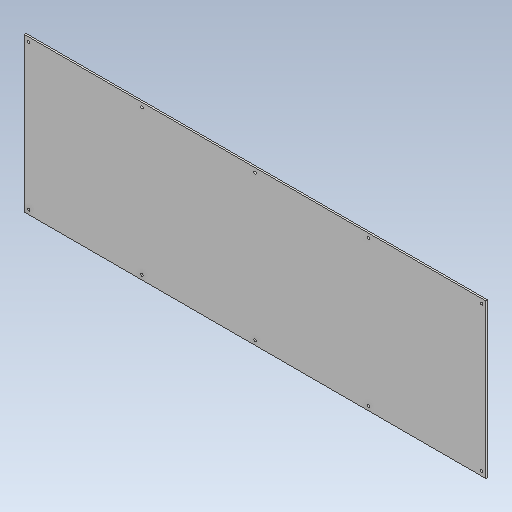
# Autodesk Inventor part: between aluminium and ferrite
Saved by Autodesk Inventor 2021 (Build 250183000, 183)
## iProperties
Created: 2022-01-22
Part Number: between aluminium and ferrite
Material: Generic
Document SubType Name: Modeling
Designer: avan411
Density: 1 g/cm^3
Appearance: Default
Author: avan411
Autodesk Inventor part; units mm, degrees
ref_plane "YZ Plane" through (0, 0, 0) normal (1, 0, 0) x (0, 1, 0)
ref_plane "XZ Plane" through (0, 0, 0) normal (0, 1, 0) x (-1, 0, 0)
ref_plane "XY Plane" through (0, 0, 0) normal (0, 0, 1) x (1, 0, 0)
sketch "Sketch1" plane through (0, 0, 0) normal (0, 0, 1) x (1, 0, 0)
  line L0 (525, 175) -> (-525, 175) projected
  line L1 (525, -175) -> (-525, -175) projected
  line L2 (-525, 175) -> (-525, -175) projected
  line L3 (525, -175) -> (525, 175) projected
  circle A0 centre (515, 165) radius 3 projected
  line L4 (525, -175) -> (-525, -175) projected
  line L5 (-525, -175) -> (-525, 175) projected
  line L6 (-525, 175) -> (525, 175) projected
  line L7 (525, 175) -> (525, -175) projected
  circle A1 centre (-515, 165) radius 3 projected
  circle A2 centre (257.5, 165) radius 3 projected
  circle A3 centre (-515, -165) radius 3 projected
  circle A4 centre (-257.5, -165) radius 3 projected
  circle A5 centre (0, -165) radius 3 projected
  circle A6 centre (257.5, -165) radius 3 projected
  circle A7 centre (515, -165) radius 3 projected
  circle A8 centre (-257.5, 165) radius 3 projected
  circle A9 centre (0, 165) radius 3 projected
  circle A10 centre (515, 165) radius 3 projected
  arc A11 (434.5, 36.45) -> (475.35, 77.3) centre (434.5, 77.3) ccw projected
  line L8 (434.5, 36.45) -> (0, 36.45) projected
  line L9 (0, 36.45) -> (0, 32.15) projected
  line L10 (0, 32.15) -> (434.5, 32.15) projected
  arc A12 (434.5, 32.15) -> (479.65, 77.3) centre (434.5, 77.3) ccw projected
  line L11 (479.65, 77.3) -> (479.65, 85.5) projected
  arc A13 (479.65, 85.5) -> (434.5, 130.65) centre (434.5, 85.5) ccw projected
  line L12 (434.5, 130.65) -> (-434.5, 130.65) projected
  arc A14 (-434.5, 130.65) -> (-479.65, 85.5) centre (-434.5, 85.5) ccw projected
  line L13 (-479.65, 85.5) -> (-479.65, 65.8667) projected
  arc A15 (-479.65, 65.8667) -> (-434.5, 20.7167) centre (-434.5, 65.8667) ccw projected
  line L14 (-434.5, 20.7167) -> (445.75, 20.7167) projected
  arc A16 (445.75, 20.7167) -> (490.9, 65.8667) centre (445.75, 65.8667) ccw projected
  line L15 (490.9, 65.8667) -> (490.9, 96.25) projected
  arc A17 (490.9, 96.25) -> (445.75, 141.4) centre (445.75, 96.25) ccw projected
  line L16 (445.75, 141.4) -> (-445.75, 141.4) projected
  arc A18 (-445.75, 141.4) -> (-490.9, 96.25) centre (-445.75, 96.25) ccw projected
  line L17 (-490.9, 96.25) -> (-490.9, 54.4333) projected
  arc A19 (-490.9, 54.4333) -> (-445.75, 9.2833) centre (-445.75, 54.4333) ccw projected
  line L18 (-445.75, 9.2833) -> (457, 9.2833) projected
  arc A20 (457, 9.2833) -> (502.15, 54.4333) centre (457, 54.4333) ccw projected
  line L19 (502.15, 54.4333) -> (502.15, 107) projected
  arc A21 (502.15, 107) -> (457, 152.15) centre (457, 107) ccw projected
  line L20 (457, 152.15) -> (-457, 152.15) projected
  arc A22 (-457, 152.15) -> (-502.15, 107) centre (-457, 107) ccw projected
  line L21 (-502.15, 107) -> (-502.15, 43) projected
  arc A23 (-502.15, 43) -> (-457, -2.15) centre (-457, 43) ccw projected
  line L22 (-457, -2.15) -> (457, -2.15) projected
  arc A24 (497.85, -43) -> (457, -2.15) centre (457, -43) ccw projected
  line L23 (497.85, -43) -> (497.85, -107) projected
  arc A25 (457, -147.85) -> (497.85, -107) centre (457, -107) ccw projected
  line L24 (457, -147.85) -> (-457, -147.85) projected
  arc A26 (-497.85, -107) -> (-457, -147.85) centre (-457, -107) ccw projected
  line L25 (-497.85, -107) -> (-497.85, -54.4333) projected
  arc A27 (-457, -13.5833) -> (-497.85, -54.4333) centre (-457, -54.4333) ccw projected
  line L26 (-457, -13.5833) -> (445.75, -13.5833) projected
  arc A28 (486.6, -54.4333) -> (445.75, -13.5833) centre (445.75, -54.4333) ccw projected
  line L27 (486.6, -54.4333) -> (486.6, -96.25) projected
  arc A29 (445.75, -137.1) -> (486.6, -96.25) centre (445.75, -96.25) ccw projected
  line L28 (445.75, -137.1) -> (-445.75, -137.1) projected
  arc A30 (-486.6, -96.25) -> (-445.75, -137.1) centre (-445.75, -96.25) ccw projected
  line L29 (-486.6, -96.25) -> (-486.6, -65.8667) projected
  arc A31 (-445.75, -25.0167) -> (-486.6, -65.8667) centre (-445.75, -65.8667) ccw projected
  line L30 (-445.75, -25.0167) -> (434.5, -25.0167) projected
  arc A32 (475.35, -65.8667) -> (434.5, -25.0167) centre (434.5, -65.8667) ccw projected
  line L31 (475.35, -65.8667) -> (475.35, -85.5) projected
  arc A33 (434.5, -126.35) -> (475.35, -85.5) centre (434.5, -85.5) ccw projected
  line L32 (434.5, -126.35) -> (-434.5, -126.35) projected
  arc A34 (-475.35, -85.5) -> (-434.5, -126.35) centre (-434.5, -85.5) ccw projected
  line L33 (-475.35, -85.5) -> (-475.35, -77.3) projected
  arc A35 (-434.5, -36.45) -> (-475.35, -77.3) centre (-434.5, -77.3) ccw projected
  line L34 (-434.5, -36.45) -> (0, -36.45) projected
  line L35 (0, -36.45) -> (0, -32.15) projected
  line L36 (0, -32.15) -> (-434.5, -32.15) projected
  arc A36 (-434.5, -32.15) -> (-479.65, -77.3) centre (-434.5, -77.3) ccw projected
  line L37 (-479.65, -77.3) -> (-479.65, -85.5) projected
  arc A37 (-479.65, -85.5) -> (-434.5, -130.65) centre (-434.5, -85.5) ccw projected
  line L38 (-434.5, -130.65) -> (434.5, -130.65) projected
  arc A38 (434.5, -130.65) -> (479.65, -85.5) centre (434.5, -85.5) ccw projected
  line L39 (479.65, -85.5) -> (479.65, -65.8667) projected
  arc A39 (479.65, -65.8667) -> (434.5, -20.7167) centre (434.5, -65.8667) ccw projected
  line L40 (434.5, -20.7167) -> (-445.75, -20.7167) projected
  arc A40 (-445.75, -20.7167) -> (-490.9, -65.8667) centre (-445.75, -65.8667) ccw projected
  line L41 (-490.9, -65.8667) -> (-490.9, -96.25) projected
  arc A41 (-490.9, -96.25) -> (-445.75, -141.4) centre (-445.75, -96.25) ccw projected
  line L42 (-445.75, -141.4) -> (445.75, -141.4) projected
  arc A42 (445.75, -141.4) -> (490.9, -96.25) centre (445.75, -96.25) ccw projected
  line L43 (490.9, -96.25) -> (490.9, -54.4333) projected
  arc A43 (490.9, -54.4333) -> (445.75, -9.2833) centre (445.75, -54.4333) ccw projected
  line L44 (445.75, -9.2833) -> (-457, -9.2833) projected
  arc A44 (-457, -9.2833) -> (-502.15, -54.4333) centre (-457, -54.4333) ccw projected
  line L45 (-502.15, -54.4333) -> (-502.15, -107) projected
  arc A45 (-502.15, -107) -> (-457, -152.15) centre (-457, -107) ccw projected
  line L46 (-457, -152.15) -> (457, -152.15) projected
  arc A46 (457, -152.15) -> (502.15, -107) centre (457, -107) ccw projected
  line L47 (502.15, -107) -> (502.15, -43) projected
  arc A47 (502.15, -43) -> (457, 2.15) centre (457, -43) ccw projected
  line L48 (457, 2.15) -> (-457, 2.15) projected
  arc A48 (-497.85, 43) -> (-457, 2.15) centre (-457, 43) ccw projected
  line L49 (-497.85, 43) -> (-497.85, 107) projected
  arc A49 (-457, 147.85) -> (-497.85, 107) centre (-457, 107) ccw projected
  line L50 (-457, 147.85) -> (457, 147.85) projected
  arc A50 (497.85, 107) -> (457, 147.85) centre (457, 107) ccw projected
  line L51 (497.85, 107) -> (497.85, 54.4333) projected
  arc A51 (457, 13.5833) -> (497.85, 54.4333) centre (457, 54.4333) ccw projected
  line L52 (457, 13.5833) -> (-445.75, 13.5833) projected
  arc A52 (-486.6, 54.4333) -> (-445.75, 13.5833) centre (-445.75, 54.4333) ccw projected
  line L53 (-486.6, 54.4333) -> (-486.6, 96.25) projected
  arc A53 (-445.75, 137.1) -> (-486.6, 96.25) centre (-445.75, 96.25) ccw projected
  line L54 (-445.75, 137.1) -> (445.75, 137.1) projected
  arc A54 (486.6, 96.25) -> (445.75, 137.1) centre (445.75, 96.25) ccw projected
  line L55 (486.6, 96.25) -> (486.6, 65.8667) projected
  arc A55 (445.75, 25.0167) -> (486.6, 65.8667) centre (445.75, 65.8667) ccw projected
  line L56 (445.75, 25.0167) -> (-434.5, 25.0167) projected
  arc A56 (-475.35, 65.8667) -> (-434.5, 25.0167) centre (-434.5, 65.8667) ccw projected
  line L57 (-475.35, 65.8667) -> (-475.35, 85.5) projected
  arc A57 (-434.5, 126.35) -> (-475.35, 85.5) centre (-434.5, 85.5) ccw projected
  line L58 (-434.5, 126.35) -> (434.5, 126.35) projected
  arc A58 (475.35, 85.5) -> (434.5, 126.35) centre (434.5, 85.5) ccw projected
  line L59 (475.35, 85.5) -> (475.35, 77.3) projected
  point P0 (0, 0)
extrude "Extrusion1" add sketch "Sketch1" along normal blind 4 contours L3 L1 L2 L0 | A11 L59 A58 L58 A57 L57 A56 L56 A55 L55 A54 L54 A53 L53 A52 L52 A51 L51 A50 L50 A49 L49 A48 L48 A47 L47 A46 L46 A45 L45 A44 L44 A43 L43 A42 L42 A41 L41 A40 L40 A39 L39 A38 L38 A37 L37 A36 L36 L35 L34 A35 L33 A34 L32 A33 L31 A32 L30 A31 L29 A30 L28 A29 L27 A28 L26 A27 L25 A26 L24 A25 L23 A24 L22 A23 L21 A22 L20 A21 L19 A20 L18 A19 L17 A18 L16 A17 L15 A16 L14 A15 L13 A14 L12 A13 L11 A12 L10 L9 L8
body "Solid1"
